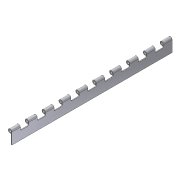
# Autodesk Inventor part: FE-00004-03A
Saved by Autodesk Inventor 2012 (Build 160160000, 160)
## iProperties
Created: 2008-05-29
Part Number: FE-00004-03A
Document SubType Name: Modeling
Designer: narosenberg
Density: 1 g/cm^3
Mass: 46.294 g
Surface Area: 442.314 cm^2
Volume: 46.294 cm^3
Material: Default
Author: narosenberg
Autodesk Inventor part; units mm, degrees
ref_plane "YZ Plane" through (0, 0, 0) normal (1, 0, 0) x (0, 1, 0)
ref_plane "XZ Plane" through (0, 0, 0) normal (0, 1, 0) x (-1, 0, 0)
ref_plane "XY Plane" through (0, 0, 0) normal (0, 0, 1) x (1, 0, 0)
sketch "Sketch1" plane through (0, 0, 0) normal (0, 0, 1) x (1, 0, 0)
  line L0 (-3.3994, 19.4704) -> (-3.3994, -14.4081)
  line L1 (-3.3994, -14.4081) -> (-5.6854, -14.4081)
  arc A0 (-3.3994, 19.4704) -> (-6.6643, 14.3475) centre (-9.0509, 19.4704) ccw
  arc A1 (-5.6854, 19.4704) -> (-7.7383, 16.3714) centre (-9.0509, 19.4704) ccw
  line L2 (-7.7383, 16.3714) -> (-6.6643, 14.3475)
  line L3 (-5.6854, -14.4081) -> (-5.6854, 19.4704)
  dimension "d0" = 11.303
  dimension "d2" = 2.286
  constraints: 8 end point, 4 point on circle, 2 centre point, 2 tangent, 1 coincident, 1 parallel
  measures "d0" diameter of A0
  measures "d2" distance between parallel lines of L0 L3
extrude "Extrusion1" add sketch "Sketch1" along normal blind 482.6
sketch "Sketch2" plane through (-3.3994, -14.4081, 0) normal (1, 0, 0) x (0, 0, -1)
  line L0 (-482.6, 33.8785) -> (-482.6, 0) projected
  line L1 (-457.2, 50.4757) -> (-431.8, 50.4757)
  line L2 (-431.8, 50.4757) -> (-431.8, 25.052)
  line L3 (-431.8, 25.052) -> (-457.2, 25.052)
  line L4 (-457.2, 25.052) -> (-457.2, 50.4757)
  line L5 (-482.6, 37.244) -> (0, 37.244) projected
  line L6 (-482.6, 33.8785) -> (-482.6, 30.7795) projected
  line L7 (0, 30.7795) -> (-482.6, 30.7795) projected
  line L8 (0, 30.7795) -> (0, 33.8785) projected
  line L9 (0, 33.8785) -> (-482.6, 33.8785) projected
  line L10 (0, 28.227) -> (-482.6, 28.227) projected
  dimension "d5" = 25.4
  dimension "d6" = 25.4
  dimension "d7" = 3.175
  constraints: 8 end point, 2 parallel, 1 horizontal, 1 perpendicular
  measures "d5" distance between parallel lines of L0 L4
  measures "d6" distance of L1.start L1.end
  measures "d7" distance between parallel lines of L3 L10
extrude "Extrusion2" cut sketch "Sketch2" against normal through all contours L9 L2 L7 L4 | L4 L5 L2 L9 | L7 L2 L10 L4 | L4 L1 L2 L5 | L10 L2 L3 L4
fillet "Fillet1" radius 3.175 2 edges at (-4.5424, 10.6439, 431.8) (-4.5424, 10.6439, 457.2)
pattern_linear "Rectangular Pattern1" count 9 spacing 50.8 along (0, 0, -1) of "Extrusion2", "Fillet1"
body "Solid1"
